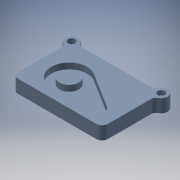
# Autodesk Inventor part: Tutorial1
Saved by Autodesk Inventor 2016 (Build 200138000, 138)
## iProperties
Created: 2012-10-25
Part Number: Tutorial1
Material: Generic
Document SubType Name: Modeling
Designer: Autodesk, Inc.
Density: 1 g/cm^3
Appearance: Light Steel Blue
Author: Autodesk, Inc.
Autodesk Inventor part; units mm, degrees
ref_plane "YZ Plane" through (0, 0, 0) normal (1, 0, 0) x (0, 1, 0)
ref_plane "XZ Plane" through (0, 0, 0) normal (0, 1, 0) x (-1, 0, 0)
ref_plane "XY Plane" through (0, 0, 0) normal (0, 0, 1) x (1, 0, 0)
sketch "Sketch1" plane through (0, 0, 0) normal (0, 0, 1) x (1, 0, 0)
  line L0 (-85.9222, 66) -> (85.9222, 66)
  line L1 (100, 51.9222) -> (100, -66)
  line L2 (100, -66) -> (-100, -66)
  line L3 (-100, -66) -> (-100, 51.9222)
  line L4 (-100, 66) -> (100, -66) construction
  line L5 (100, 66) -> (-100, -66) construction
  arc A0 (-85.9222, 66) -> (-100, 51.9222) centre (-100, 66) ccw
  arc A1 (100, 51.9222) -> (85.9222, 66) centre (100, 66) ccw
  line L6 (0, 116.2908) -> (0, -96.3818) projected
  line L7 (-167.8726, 0) -> (167.8726, 0) projected
  point P0 (0, 0)
  dimension "d0" = 200
  dimension "d1" = 132
  dimension "d3" = 28.1556
  dimension "d35" = 200
  constraints: 12 end point, 4 point on circle, 2 centre point, 2 coincident, 2 midpoint, 2 parallel, 1 equal radius, 1 horizontal, 1 perpendicular, 1 symmetric about line, 2 other
  measures "d0" distance of L1.end L2.end
  measures "d1" distance of L5.start L1.end
  measures "d3" diameter of A1
  measures "d35" distance of L5.start L4.start
extrude "Extrusion1" add sketch "Sketch1" along normal blind 29.2
fillet "Fillet1" radius 12 6 edges at (-85.9222, 66, 14.6) (85.9222, 66, 14.6) (-100, 51.9222, 14.6) (-100, -66, 14.6) (100, -66, 14.6) (100, 51.9222, 14.6)
sketch "Sketch2" plane through (0, 0, 29.2) normal (0, 0, 1) x (1, 0, 0)
  arc A0 (-87.5012, 72.4781) -> (-106.4781, 53.5012) centre (-100, 66) ccw projected
  circle A1 centre (-33.4, -6) radius 21.33
  arc A2 (-12.2198, 27.9323) -> (-33.4, -46) centre (-33.4, -6) ccw
  arc A3 (59.8, -46) -> (66.8424, -21.4175) centre (59.8, -32.7) ccw
  line L0 (-33.4, -46) -> (59.8, -46)
  line L1 (66.8424, -21.4175) -> (-12.2198, 27.9323)
  point P0 (-88, -66)
  point P1 (0, 0)
  dimension "d7" = 42.66
  dimension "d8" = 60
  dimension "d9" = 66.6
  dimension "d10" = 80
  dimension "d12" = 93.2
  dimension "d13" = 26.6
  constraints: 4 end point, 4 point on circle, 4 tangent, 3 centre point, 1 coincident, 1 horizontal
  measures "d7" diameter of A1
  measures "d8" vertical distance of A1.centre point (-88, -66)
  measures "d9" horizontal distance of A1.centre A0.centre
  measures "d10" diameter of A2
  measures "d12" horizontal distance of A3.centre A1.centre
  measures "d13" diameter of A3
extrude "Extrusion2" cut sketch "Sketch2" against normal blind 13.2
hole "Hole1" at (-100, 66, 29.2) direction (0, 0, -1) diameter 5 end through all counterbore diameter 16 counterbore depth 13.2
hole "Hole2" at (100, 66, 29.2) direction (0, 0, -1) diameter 5 end through all counterbore diameter 16 counterbore depth 10
equation "\"d1\" = 0.66 * d0"
equation "\"d3\" = 0.2133 * d1"
equation "\"d35\" = d0"
equation "\"d4\" = 0.146 * d0"
equation "\"d6\" = 0.06 * d0"
equation "\"d7\" = 0.2133 * d0"
equation "\"d8\" = 0.3 * d0"
equation "\"d9\" = 0.333 * d0"
equation "\"d10\" = 0.4 * d0"
equation "\"d12\" = 0.466 * d0"
equation "\"d13\" = 0.133 * d0"
equation "\"d15\" = 0.066 * d0"
equation "\"d21\" = 0.08 * d0"
equation "\"d22\" = 0.066 * d0"
equation "\"d30\" = 0.08 * d0"
equation "\"d31\" = 0.05 * d0"
body "Solid1"
